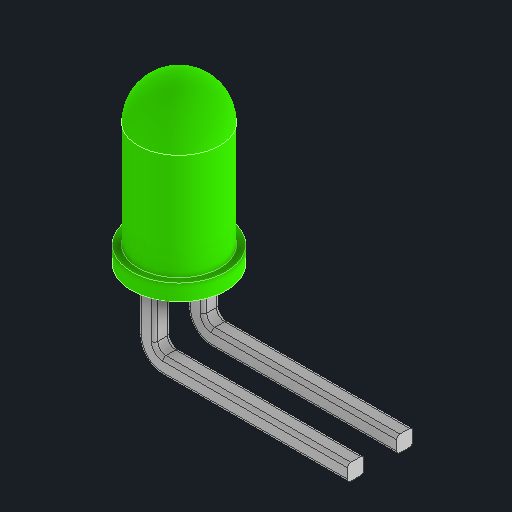
# Autodesk Inventor part: P_LED_5
Saved by Autodesk Inventor 2026 (Build 300175000, 175)
## iProperties
Created: 2025-09-04
Part Number: P_LED_5
Material: Generisch
Document SubType Name: Modeling
Designer: FAL
Density: 1 g/cm^3
Appearance: Vorgabe
Author: FAL
Autodesk Inventor part; units mm, degrees
ref_plane "YZ Plane" through (0, 0, 0) normal (1, 0, 0) x (0, 1, 0)
sketch "Skizze1" plane through (0, 0, 0) normal (0, 0, 1) x (1, 0, 0)
  circle A0 centre (0, 0) radius 2.9
  dimension "d0" = 5.8
  constraints: 1 centre point, 1 coincident
  measures "d0" diameter of A0
extrude "Extrusion1" add sketch "Skizze1" along normal blind 1
sketch "Skizze2" plane through (0, 0, 1) normal (0, 0, 1) x (1, 0, 0)
  circle A0 centre (0, 0) radius 2.5
  dimension "d3" = 5
  constraints: 1 centre point, 1 coincident
  measures "d3" diameter of A0
extrude "Extrusion2" add sketch "Skizze2" along normal blind 9
fillet "Rundung1" radius 2.5 1 edges at (-2.5, 0, 10)
sketch "Skizze3" plane through (0, 0, 0) normal (0, 0, -1) x (-1, 0, 0)
  point P0 (0, 0)
ref_plane "Arbeitsebene1" through (0, -1.5, 0) normal (0, 1, 0) x (-1, 0, 0)
sketch "Skizze4" plane through (0, -1.5, 0) normal (0, 1, 0) x (-1, 0, 0)
  line L0 (0, 1.0632) -> (0, -3)
  line L1 (-1, -4) -> (-12.3472, -4)
  arc A0 (-1, -4) -> (0, -3) centre (-1, -3) ccw
  line L2 (2.9, 0) -> (-2.9, 0) projected
  point P0 (0, 0)
  dimension "d8" = 1
  dimension "d9" = 4
  constraints: 4 end point, 2 point on circle, 2 tangent, 1 centre point, 1 perpendicular, 1 vertical
  measures "d8" radius of A0
  measures "d9" distance between parallel lines of L1 L2
ref_plane "Arbeitsebene2" through (12.3472, -1.5, -4) normal (1, 0, 0) x (0, 1, 0)
sketch "Skizze5" plane through (12.3472, -1.5, -4) normal (1, 0, 0) x (0, 1, 0)
  line L0 (0.5, -0.5) -> (-0.5, -0.5)
  line L1 (-0.5, -0.5) -> (-0.5, 0.5)
  line L2 (-0.5, 0.5) -> (0.5, 0.5)
  line L3 (0.5, 0.5) -> (0.5, -0.5)
  line L4 (0.5, -0.5) -> (-0.5, 0.5) construction
  line L5 (-0.5, -0.5) -> (0.5, 0.5) construction
  point P0 (1.5, 4)
  point P1 (0, 0)
  dimension "d10" = 1
  constraints: 12 end point, 2 midpoint, 2 parallel, 2 perpendicular, 1 horizontal
  measures "d10" distance of L0.end L1.end
sweep "Sweeping1" add profiles "Skizze5" path "Skizze4" separate body path curves L1 A0 L0
fillet "Rundung2" radius 0.2 12 edges at (-0.5, -2, -0.9684) (-0.0607, -2, -4.0607) (6.6736, -2, -4.5) (0.5, -2, -0.9684) (0.6464, -2, -3.3536) (6.6736, -2, -3.5) (-0.5, -1, -0.9684) (-0.0607, -1, -4.0607) (6.6736, -1, -4.5) (0.5, -1, -0.9684) (0.6464, -1, -3.3536) (6.6736, -1, -3.5)
mirror "Spiegeln1" about plane through (0, 0, 0) normal (0, 1, 0) bodies 2
